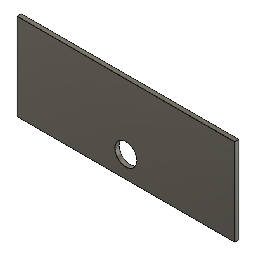
Table_17p1_Problem_8 (Autodesk Fusion 360 design; units mm, degrees)
Autodesk Fusion 360 part; units mm, degrees
sketch "Sketch1" plane through (0, 0, 0) normal (0, 0, 1) x (1, 0, 0)
  line L0 (-250, 100) -> (250, 100)
  line L1 (250, 100) -> (250, -100)
  line L2 (250, -100) -> (-250, -100)
  line L3 (-250, -100) -> (-250, 100)
  line L4 (250, 0) -> (-250, 0) construction
  line L5 (0, 100) -> (0, -100) construction
  circle A0 centre (0, -50) radius 25
  dimension "Total_Width" = 500
  dimension "Total_Height" = 200
  dimension "Hole_Radius" = 25
  dimension "Hole_Offset" = 50
  constraint horizontal L0
  constraint vertical L1
  constraint horizontal L2
  constraint vertical L3
  constraint midpoint L1 L4.start
  constraint coincident L3 L4.end
  constraint midpoint L0 L5.start
  constraint coincident L2 L5.end
  constraint vertical L5
  constraint horizontal L4
  constraint coincident origin L4
  constraint coincident origin L5
  constraint coincident L5 A0.centre
  measures "Total_Width" distance of L0.start L0.end
  measures "Total_Height" distance of L0.end L1.end
  measures "Hole_Radius" radius of A0
  measures "Hole_Offset" distance of L4 A0.centre
extrude "Extrude1" add sketch "Sketch1" along normal mid plane 10
equation "Thickness = 1 cm"
